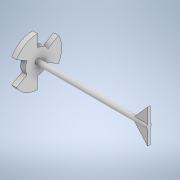
# Autodesk Inventor part: Powder Arrow
Saved by Autodesk Inventor 2021 (Build 250183000, 183)
## iProperties
Created: 2021-01-08
Part Number: Powder Arrow
Material: Generic
Document SubType Name: Modeling
Designer: saipr
Density: 1 g/cm^3
Appearance: Default
Author: saipr
Autodesk Inventor part; units mm, degrees
ref_plane "YZ Plane" through (0, 0, 0) normal (1, 0, 0) x (0, 1, 0)
ref_plane "XZ Plane" through (0, 0, 0) normal (0, 1, 0) x (-1, 0, 0)
ref_plane "XY Plane" through (0, 0, 0) normal (0, 0, 1) x (1, 0, 0)
sketch "Sketch1" plane through (0, 0, 0) normal (0, 0, 1) x (1, 0, 0)
  line L0 (-152.4, 6.35) -> (152.4, 6.35)
  line L1 (152.4, 6.35) -> (152.4, -6.35)
  line L2 (152.4, -6.35) -> (-152.4, -6.35)
  line L3 (-152.4, -6.35) -> (-152.4, 6.35)
  line L4 (-152.4, 6.35) -> (152.4, -6.35) construction
  line L5 (152.4, 6.35) -> (-152.4, -6.35) construction
  line L6 (-152.4, 0) -> (-146.05, 0)
  line L7 (-152.4, -31.75) -> (-139.7, -31.75)
  line L8 (-139.7, -31.75) -> (-139.7, 31.75)
  line L9 (-139.7, 31.75) -> (-152.4, 31.75)
  line L10 (-152.4, 31.75) -> (-152.4, -31.75)
  line L11 (-152.4, -31.75) -> (-139.7, 31.75) construction
  line L12 (-139.7, -31.75) -> (-152.4, 31.75) construction
  line L13 (-152.4, 0) -> (-165.1, 0)
  line L14 (-165.1, 0) -> (-152.4, 6.35)
  line L15 (152.4, 0) -> (152.4, 44.45)
  line L16 (152.4, 44.45) -> (113.1983, 0)
  line L17 (-146.05, 0) -> (152.4, 0)
  line L18 (152.4, 0) -> (152.4, -44.45)
  line L19 (152.4, -44.45) -> (113.1983, 0)
  point P0 (0, 0)
  point P1 (-139.7, 6.35)
  dimension "d0" = 304.8
  dimension "d1" = 12.7
  dimension "d2" = 6.35
  dimension "d3" = 12.7
  dimension "d4" = 63.5
  dimension "d5" = 12.7
  dimension "d6" = 44.45
  dimension "d8" = 41.41
  constraints: 40 end point, 6 midpoint, 5 horizontal, 4 parallel, 2 perpendicular, 2 symmetric about line, 1 point on line, 1 vertical
  measures "d0" distance of L1.end L2.end
  measures "d1" distance of L0.end L1.end
  measures "d2" distance of L6.start L6.end
  measures "d3" distance of L9.end L8.end
  measures "d4" distance of L8.end L7.end
  measures "d5" distance of L6.start L13.end
  measures "d6" distance of L15.start L15.end
  measures "d8" angle of L16 L15
revolve "Revolution1" add sketch "Sketch1" angle 360 about axis through (-146.05, 0, 0) along (1, 0, 0) contours L10 L9 L8 L0 | L0 L8 L17 L6 L3 | L3 L13 L14 | L0 L16 L17 L8 | L0 L1 L17 L16
extrude "Extrusion1" add sketch "Sketch1" along normal mid plane 6.35 contours L16 L15 L0 | L0 L1 L17 L16 | L17 L1 L2 L19 | L2 L18 L19
sketch "Sketch2" plane through (-139.7, 0, 0) normal (1, 0, 0) x (0, 0, -1)
  circle A0 centre (0, 0) radius 63.5
  circle A1 centre (0, 0) radius 6.35
  line L0 (0, 0) -> (0, 63.5)
  line L1 (0, 0) -> (54.9926, -31.75)
  line L2 (0, 0) -> (-54.9926, -31.75)
  line L3 (0, 0) -> (54.9926, 31.75)
  line L4 (0, 0) -> (0, -63.5)
  line L5 (0, 0) -> (-54.9926, 31.75)
  circle A2 centre (0, 0) radius 31.75
  point P0 (0, -31.75)
  point P1 (-27.4963, -15.875)
  point P2 (27.4963, 15.875)
  point P3 (27.4963, -15.875)
  point P4 (-27.4963, 15.875)
  point P5 (0, 31.75)
  dimension "d12" = 12.7
  dimension "d13" = 120
  dimension "d14" = 120
  dimension "d15" = 60
  dimension "d16" = 60
  constraints: 12 end point, 6 point on circle, 3 centre point, 3 coincident, 2 vertical
  measures "d12" diameter of A1
  measures "d13" angle of L1 L0
  measures "d14" angle of L2 L0
  measures "d15" angle of L3 L0
  measures "d16" angle of L2 L5
extrude "Extrusion2" add sketch "Sketch2" against normal blind 12.7 contours A0 L1 A2 L3 | L0 A2 L5 A0 | A0 L2 A2 L4
body "Solid1"
